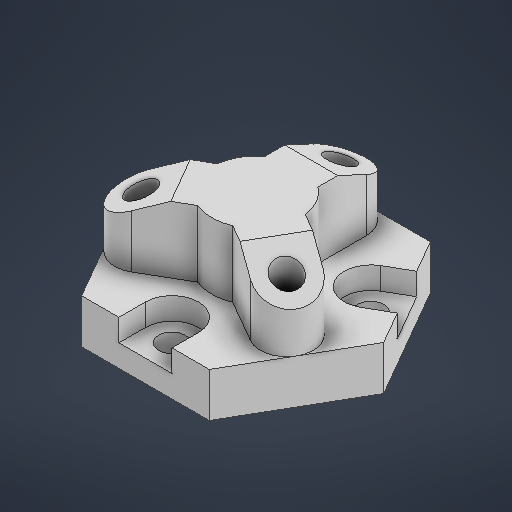
# Autodesk Inventor part: b3
Saved by Autodesk Inventor 2025.4 (Build 294407000, 407)
## iProperties
Created: 2026-05-15
Part Number: b3
Material: Generic
Document SubType Name: Modeling
Designer: VuQuan
Density: 1 g/cm^3
Appearance: Default
Author: VuQuan
Autodesk Inventor part; units mm, degrees
ref_plane "YZ Plane" through (0, 0, 0) normal (1, 0, 0) x (0, 1, 0)
ref_plane "XZ Plane" through (0, 0, 0) normal (0, 1, 0) x (-1, 0, 0)
ref_plane "XY Plane" through (0, 0, 0) normal (0, 0, 1) x (1, 0, 0)
sketch "Sketch1" plane through (0, 0, 0) normal (0, 1, 0) x (-1, 0, 0)
  line L0 (57.735, 0) -> (43.3013, -25)
  line L1 (0, 50) -> (28.8675, 50)
  line L2 (28.8675, 50) -> (57.735, 0)
  line L3 (0, 0) -> (0, 50)
  line L4 (0, 0) -> (57.735, 0) construction
  line L5 (0, 0) -> (43.3013, 25) construction
  line L6 (0, 0) -> (43.3013, -25)
  line L7 (12, 50) -> (12, 38)
  arc A0 (0, 26) -> (12, 38) centre (0, 38) ccw
  arc A1 (0, 32) -> (0, 44) centre (0, 38) ccw
  arc A2 (17.3205, -10) -> (19.8564, -2.3923) centre (0, 0) ccw
  line L8 (49.3013, -14.6077) -> (38.909, -8.6077)
  arc A3 (38.909, -8.6077) -> (22.5167, -13) centre (32.909, -19) ccw
  arc A4 (38.1051, -22) -> (27.7128, -16) centre (32.909, -19) ccw
  line L9 (19.8564, -2.3923) -> (38.909, 8.6077)
  arc A5 (38.909, 8.6077) -> (26.909, 29.3923) centre (32.909, 19) ccw
  line L10 (26.909, 29.3923) -> (7.8564, 18.3923)
  circle A6 centre (32.909, 19) radius 6
  arc A7 (7.8564, 18.3923) -> (0, 20) centre (0, 0) ccw
  arc A8 (19.8564, -2.3923) -> (7.8564, 18.3923) centre (0, 0) ccw construction
  point P0 (27.7128, -16)
  point P1 (22.5167, -13)
  dimension "d1" = 100
  dimension "d2" = 24
  dimension "d3" = 38
  dimension "d4" = 6
  dimension "d5" = 20
  constraints: 22 end point, 17 point on circle, 9 centre point, 8 point on line, 7 symmetric about line, 5 coincident, 4 tangent, 2 equal radius, 2 horizontal, 2 parallel, 2 vertical, 1 midpoint, 1 vertical alignment, 6 other
  measures "d1" diameter of L1 L4
  measures "d2" diameter of L7 L3
  measures "d3" distance of point (0, 0) A0.centre
  measures "d4" radius of A1
  measures "d5" radius of A2
extrude "Extrusion1" add sketch "Sketch1" along normal blind 20 contours L0 L8 A3 L6 A2 L9 A5 L2 | L0 L6 A4 A3 L8 | A5 L10 A7 L3 A0 L7 L1 L2 | A5 L9 A2 L6 L3 A7 L10 | L6 A4 | L7 A0 L3 A1 L1 | A1 L3 | A6
extrude "Extrusion2" cut sketch "Sketch1" along normal up to surface (20 mm away) contours L6 A4 | A1 L3
extrude "Extrusion3" cut sketch "Sketch1" against normal blind 10 from surface at 20 contours L0 L6 A4 A3 L8 | L7 A0 L3 A1 L1
extrude "Extrusion4" add sketch "Sketch1" along normal blind 50 contours A5 L9 A2 L6 L3 A7 L10
sketch "Sketch2" plane through (-7.8564, 20, 18.3923) normal (0.5, 0, 0.8660254) x (0.8660254, 0, -0.5)
  line L0 (-22, 30) -> (0, 30) projected
  line L1 (-34, 18.3423) -> (-9, 30)
  line L2 (-34, 0) -> (-34, 30) projected
  line L3 (-9, 30) -> (-34, 30)
  line L4 (-34, 30) -> (-34, 18.3423)
  point P0 (16, -20)
  point P1 (16, 30)
  dimension "d15" = 25
  dimension "d16" = 25
  constraints: 6 end point, 2 point on line, 1 collinear
  measures "d15" distance of point (16, 30) L1.end
  measures "d16" angle of L0 L1
extrude "Extrusion5" cut sketch "Sketch2" against normal up to surface (24 mm away)
pattern_circular "Circular Pattern1" count 3 over 360 about axis through (0, 0, 0) along (0, 1, 0)
body "Solid1"
